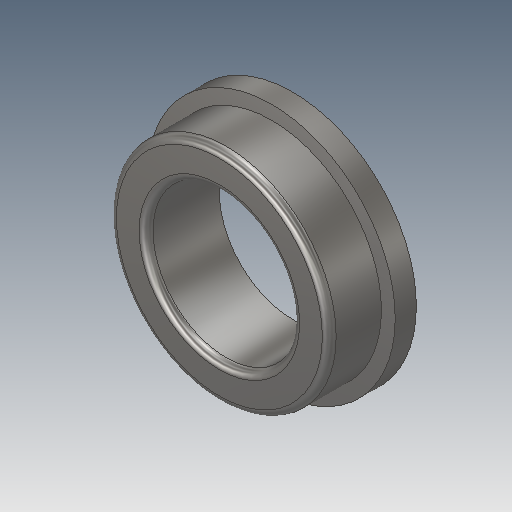
# Autodesk Inventor part: FR168ZZ flangde bearing
Saved by Autodesk Inventor 2019 (Build 230136000, 136)
## iProperties
Created: 2018-10-28
Part Number: FR168ZZ flangde bearing
Material: Steel, Alloy
Document SubType Name: Modeling
Designer: LillaHunden
Density: 7.73 g/cm^3
Appearance: Semi-Polished
Mass: 1.09824 g
Surface Area: 2.72494 cm^2
Volume: 0.142075 cm^3
Author: LillaHunden
Autodesk Inventor part; units mm, degrees
ref_plane "YZ Plane" through (0, 0, 0) normal (1, 0, 0) x (0, 1, 0)
ref_plane "XZ Plane" through (0, 0, 0) normal (0, 1, 0) x (-1, 0, 0)
ref_plane "XY Plane" through (0, 0, 0) normal (0, 0, 1) x (1, 0, 0)
sketch "Sketch1" plane through (0, 0, 0) normal (0, 0, 1) x (1, 0, 0)
  circle A0 centre (0, 0) radius 5.3595
  dimension "d0" = 10.719
  constraints: 1 centre point, 1 coincident
  measures "d0" diameter of A0
extrude "Extrusion1" add sketch "Sketch1" along normal blind 0.914
sketch "Sketch2" plane through (0, 0, 0.914) normal (0, 0, 1) x (1, 0, 0)
  circle A0 centre (0, 0) radius 4.7625
  dimension "d3" = 9.525
  constraints: 1 centre point, 1 coincident
  measures "d3" diameter of A0
extrude "Extrusion2" add sketch "Sketch2" along normal blind 3.175 from surface at -0.914
sketch "Sketch3" plane through (0, 0, 3.175) normal (0, 0, 1) x (1, 0, 0)
  circle A0 centre (0, 0) radius 3.175
  dimension "d6" = 6.35
  constraints: 1 centre point, 1 coincident
  measures "d6" diameter of A0
extrude "Extrusion3" cut sketch "Sketch3" against normal through all
fillet "Fillet1" radius 0.3 2 edges at (-4.7625, 0, 3.175) (-3.175, 0, 3.175)
body "Solid1"
